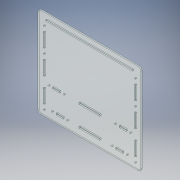
# Autodesk Inventor part: Tapa_Trasera
Saved by Autodesk Inventor 2019 (Build 230136000, 136)
## iProperties
Created: 2020-04-07
Part Number: Tapa_Trasera
Material: Generic
Document SubType Name: Modeling
Designer: Jurgen
Density: 1 g/cm^3
Appearance: Clear
Author: Jurgen
Autodesk Inventor part; units mm, degrees
ref_plane "YZ Plane" through (0, 0, 0) normal (1, 0, 0) x (0, 1, 0)
ref_plane "XZ Plane" through (0, 0, 0) normal (0, 1, 0) x (-1, 0, 0)
ref_plane "XY Plane" through (0, 0, 0) normal (0, 0, 1) x (1, 0, 0)
sketch "Sketch1" plane through (0, 0, 0) normal (0, 0, 1) x (1, 0, 0)
  line L0 (0, 40) -> (0, 0)
  line L1 (0, 40) -> (3.5, 40)
  line L2 (3.5, 40) -> (3.5, 0)
  line L3 (0, 0) -> (3.5, 0)
  line L4 (0, 57) -> (3.5, 57)
  line L5 (3.5, 53) -> (0, 53)
  line L6 (0, -13) -> (3.5, -13)
  line L7 (3.5, -17) -> (0, -17)
  line L8 (0, -30) -> (0, -70)
  line L9 (0, -30) -> (3.5, -30)
  line L10 (3.5, -30) -> (3.5, -70)
  line L11 (0, -70) -> (3.5, -70)
  line L12 (0, -100) -> (0, -140)
  line L13 (3.5, -100) -> (3.5, -140)
  line L14 (0, -100) -> (3.5, -100)
  line L15 (0, -140) -> (3.5, -140)
  line L16 (0, -153) -> (3.5, -153)
  line L17 (3.5, -157) -> (0, -157)
  line L18 (263.5, 57.0001) -> (267, 57.0001)
  line L19 (267, 53.0001) -> (263.5, 53.0001)
  line L20 (263.5, 40.0001) -> (267, 40.0001)
  line L21 (263.5, 40.0001) -> (263.5, 0.0001)
  line L22 (267, 40.0001) -> (267, 0.0001)
  line L23 (263.5, 0.0001) -> (267, 0.0001)
  line L24 (263.5, -12.9999) -> (267, -12.9999)
  line L25 (267, -16.9999) -> (263.5, -16.9999)
  line L26 (263.5, -29.9999) -> (267, -29.9999)
  line L27 (263.5, -29.9999) -> (263.5, -69.9999)
  line L28 (267, -29.9999) -> (267, -69.9999)
  line L29 (263.5, -69.9999) -> (267, -69.9999)
  line L30 (263.5, -99.9999) -> (263.5, -139.9999)
  line L31 (263.5, -99.9999) -> (267, -99.9999)
  line L32 (267, -99.9999) -> (267, -139.9999)
  line L33 (263.5, -139.9999) -> (267, -139.9999)
  line L34 (263.5, -152.9999) -> (267, -152.9999)
  line L35 (267, -156.9999) -> (263.5, -156.9999)
  line L36 (23.5, -149.9999) -> (23.5, -144.9999)
  line L37 (27.5, -144.9999) -> (27.5, -149.9999)
  line L38 (37.5, -144.9999) -> (37.5, -149.9999)
  line L39 (57.5, -144.9999) -> (57.5, -149.9999)
  line L40 (67.5, -149.9999) -> (67.5, -144.9999)
  line L41 (71.5, -144.9999) -> (71.5, -149.9999)
  line L42 (37.5, -144.9999) -> (57.5, -144.9999)
  line L43 (57.5, -149.9999) -> (37.5, -149.9999)
  line L44 (103.5, -144.9999) -> (103.5, -149.9999)
  line L45 (103.5, -144.9999) -> (163.5, -144.9999)
  line L46 (163.5, -149.9999) -> (103.5, -149.9999)
  line L47 (163.5, -144.9999) -> (163.5, -149.9999)
  line L48 (195.5, -149.9999) -> (195.5, -144.9999)
  line L49 (199.5, -144.9999) -> (199.5, -149.9999)
  line L50 (209.5, -144.9999) -> (209.5, -149.9999)
  line L51 (229.5, -144.9999) -> (229.5, -149.9999)
  line L52 (209.5, -144.9999) -> (229.5, -144.9999)
  line L53 (229.5, -149.9999) -> (209.5, -149.9999)
  line L54 (239.5, -149.9999) -> (239.5, -144.9999)
  line L55 (243.5, -144.9999) -> (243.5, -149.9999)
  line L56 (253.5, -84.9999) -> (253.5, -89.9999)
  line L57 (249.5, -89.9999) -> (249.5, -84.9999)
  line L58 (239.5, -84.9999) -> (239.5, -89.9999)
  line L59 (239.5, -84.9999) -> (219.5, -84.9999)
  line L60 (219.5, -84.9999) -> (219.5, -89.9999)
  line L61 (239.5, -89.9999) -> (219.5, -89.9999)
  line L62 (205.5, -89.9999) -> (205.5, -84.9999)
  line L63 (209.5, -84.9999) -> (209.5, -89.9999)
  line L64 (103.5, -84.9999) -> (163.5, -84.9999)
  line L65 (163.5, -89.9999) -> (103.5, -89.9999)
  line L66 (163.5, -84.9999) -> (163.5, -89.9999)
  line L67 (103.5, -84.9999) -> (103.5, -89.9999)
  line L68 (57.5, -89.9999) -> (57.5, -84.9999)
  line L69 (61.5, -84.9999) -> (61.5, -89.9999)
  line L70 (47.5, -84.9999) -> (47.5, -89.9999)
  line L71 (27.5, -84.9999) -> (47.5, -84.9999)
  line L72 (47.5, -89.9999) -> (27.5, -89.9999)
  line L73 (27.5, -84.9999) -> (27.5, -89.9999)
  line L74 (13.5, -89.9999) -> (13.5, -84.9999)
  line L75 (17.5, -84.9999) -> (17.5, -89.9999)
  line L76 (-15, 82) -> (-15, -161.9999)
  arc A0 (-7, 90) -> (-15, 82) centre (-7, 82) ccw
  line L77 (274, 90) -> (-7, 90)
  arc A1 (282, 82) -> (274, 90) centre (274, 82) ccw
  line L78 (282, -161.9999) -> (282, 82)
  arc A2 (-15, -161.9999) -> (-7, -169.9999) centre (-7, -161.9999) ccw
  line L79 (-7, -169.9999) -> (274, -169.9999)
  arc A3 (274, -169.9999) -> (282, -161.9999) centre (274, -161.9999) ccw
  line L80 (1.75, 57) -> (1.75, 53)
  line L81 (1.75, -13) -> (1.75, -17)
  line L82 (1.75, -153) -> (1.75, -157)
  line L83 (23.5, -147.4999) -> (27.5, -147.4999)
  line L84 (67.5, -147.4999) -> (71.5, -147.4999)
  line L85 (195.5, -147.4999) -> (199.5, -147.4999)
  line L86 (239.5, -147.4999) -> (243.5, -147.4999)
  line L87 (265.25, -156.9999) -> (265.25, -152.9999)
  line L88 (13.5, -87.4999) -> (17.5, -87.4999)
  line L89 (57.5, -87.4999) -> (61.5, -87.4999)
  line L90 (205.5, -87.4999) -> (209.5, -87.4999)
  line L91 (249.5, -87.4999) -> (253.5, -87.4999)
  line L92 (265.25, -16.9999) -> (265.25, -12.9999)
  line L93 (265.25, 53.0001) -> (265.25, 57.0001)
  circle A4 centre (1.75, 55) radius 2
  circle A5 centre (1.75, -15) radius 2
  circle A6 centre (1.75, -155) radius 2
  circle A7 centre (25.5, -147.4999) radius 2
  circle A8 centre (69.5, -147.4999) radius 2
  circle A9 centre (197.5, -147.4999) radius 2
  circle A10 centre (241.5, -147.4999) radius 2
  circle A11 centre (265.25, -154.9999) radius 2
  circle A12 centre (15.5, -87.4999) radius 2
  circle A13 centre (59.5, -87.4999) radius 2
  circle A14 centre (207.5, -87.4999) radius 2
  circle A15 centre (251.5, -87.4999) radius 2
  circle A16 centre (265.25, -14.9999) radius 2
  circle A17 centre (265.25, 55.0001) radius 2
  constraints: 188 end point, 42 midpoint, 8 horizontal alignment, 8 point on circle, 7 centre point, 3 tangent, 3 vertical alignment, 22 other
extrude "Extrusion1" add sketch "Sketch1" along normal blind 3.5
sketch "Sketch2" plane through (0, 0, 3.5) normal (0, 0, 1) x (1, 0, 0)
  line L0 (163.5, -84.9999) -> (163.5, -89.9999) construction
  line L1 (163.5, -89.9999) -> (103.5, -89.9999) construction
  line L2 (103.5, -89.9999) -> (103.5, -84.9999) construction
  line L3 (103.5, -84.9999) -> (163.5, -84.9999) construction
  line L4 (103.5, -144.9999) -> (163.5, -144.9999) construction
  line L5 (163.5, -144.9999) -> (163.5, -149.9999) construction
  line L6 (163.5, -149.9999) -> (103.5, -149.9999) construction
  line L7 (103.5, -149.9999) -> (103.5, -144.9999) construction
  line L8 (263.5, -99.9999) -> (267, -99.9999) construction
  line L9 (267, -99.9999) -> (267, -139.9999) construction
  line L10 (267, -139.9999) -> (263.5, -139.9999) construction
  line L11 (263.5, -139.9999) -> (263.5, -99.9999) construction
  line L12 (267, -29.9999) -> (267, -69.9999) construction
  line L13 (267, -69.9999) -> (263.5, -69.9999) construction
  line L14 (263.5, -69.9999) -> (263.5, -29.9999) construction
  line L15 (263.5, -29.9999) -> (267, -29.9999) construction
  line L16 (267, 40.0001) -> (267, 0.0001) construction
  line L17 (267, 0.0001) -> (263.5, 0.0001) construction
  line L18 (263.5, 0.0001) -> (263.5, 40.0001) construction
  line L19 (263.5, 40.0001) -> (267, 40.0001) construction
  line L20 (0, -100) -> (3.5, -100) construction
  line L21 (3.5, -100) -> (3.5, -140) construction
  line L22 (3.5, -140) -> (0, -140) construction
  line L23 (0, -140) -> (0, -100) construction
  line L24 (0, -30) -> (3.5, -30) construction
  line L25 (3.5, -30) -> (3.5, -70) construction
  line L26 (3.5, -70) -> (0, -70) construction
  line L27 (0, -70) -> (0, -30) construction
  line L28 (0, 40) -> (3.5, 40) construction
  line L29 (3.5, 40) -> (3.5, 0) construction
  line L30 (3.5, 0) -> (0, 0) construction
  line L31 (0, 0) -> (0, 40) construction
  line L32 (47.5, -89.9999) -> (27.5, -89.9999) construction
  line L33 (27.5, -89.9999) -> (27.5, -84.9999) construction
  line L34 (27.5, -84.9999) -> (47.5, -84.9999) construction
  line L35 (47.5, -84.9999) -> (47.5, -89.9999) construction
  line L36 (239.5, -89.9999) -> (219.5, -89.9999) construction
  line L37 (219.5, -89.9999) -> (219.5, -84.9999) construction
  line L38 (219.5, -84.9999) -> (239.5, -84.9999) construction
  line L39 (239.5, -84.9999) -> (239.5, -89.9999) construction
  line L40 (209.5, -144.9999) -> (229.5, -144.9999) construction
  line L41 (229.5, -144.9999) -> (229.5, -149.9999) construction
  line L42 (229.5, -149.9999) -> (209.5, -149.9999) construction
  line L43 (209.5, -149.9999) -> (209.5, -144.9999) construction
  line L44 (37.5, -144.9999) -> (57.5, -144.9999) construction
  line L45 (57.5, -144.9999) -> (57.5, -149.9999) construction
  line L46 (57.5, -149.9999) -> (37.5, -149.9999) construction
  line L47 (37.5, -149.9999) -> (37.5, -144.9999) construction
  circle A0 centre (265.25, 55.0001) radius 2 construction
  circle A1 centre (265.25, -14.9999) radius 2 construction
  circle A2 centre (251.5, -87.4999) radius 2 construction
  circle A3 centre (207.5, -87.4999) radius 2 construction
  circle A4 centre (59.5, -87.4999) radius 2 construction
  circle A5 centre (15.5, -87.4999) radius 2 construction
  circle A6 centre (265.25, -154.9999) radius 2 construction
  circle A7 centre (241.5, -147.4999) radius 2 construction
  circle A8 centre (197.5, -147.4999) radius 2 construction
  circle A9 centre (69.5, -147.4999) radius 2 construction
  circle A10 centre (25.5, -147.4999) radius 2 construction
  circle A11 centre (1.75, -155) radius 2 construction
  circle A12 centre (1.75, -15) radius 2 construction
  circle A13 centre (1.75, 55) radius 2 construction
  line L48 (-15, 82) -> (-15, -161.9999) construction
  arc A14 (-15, -161.9999) -> (-7, -169.9999) centre (-7, -161.9999) ccw construction
  line L49 (-7, -169.9999) -> (274, -169.9999) construction
  arc A15 (274, -169.9999) -> (282, -161.9999) centre (274, -161.9999) ccw construction
  line L50 (282, -161.9999) -> (282, 82) construction
  arc A16 (282, 82) -> (274, 90) centre (274, 82) ccw construction
  line L51 (274, 90) -> (-7, 90) construction
  arc A17 (-7, 90) -> (-15, 82) centre (-7, 82) ccw construction
  line L52 (-15, 82) -> (-15, 90) construction
  line L53 (-15, 90) -> (-7, 90) construction
  line L54 (-15.8616, 90) -> (7.6384, 90) construction
  line L55 (7.6384, 90) -> (7.6384, 73.5) construction
  line L56 (7.6384, 73.5) -> (-15.8616, 73.5) construction
  line L57 (-15.8616, 73.5) -> (-15.8616, 90) construction
  line L58 (7.6384, 73.5) -> (257.6384, 73.5)
  line L59 (257.6384, 73.5) -> (257.6384, 70)
  line L60 (257.6384, 70) -> (7.6384, 70)
  line L61 (7.6384, 70) -> (7.6384, 73.5)
  dimension "d2" = 23.5
  dimension "d3" = 16.5
  dimension "d4" = 250
  dimension "d5" = 3.5
  constraints: 20 end point, 4 parallel, 3 perpendicular, 2 horizontal, 1 tangent, 1 vertical
  measures "d2" distance of L55.end L56.end
  measures "d3" distance of L54.end L55.end
  measures "d4" distance of L59.end L60.end
  measures "d5" distance of L58.end L59.end
extrude "Extrusion2" cut sketch "Sketch2" against normal blind 3.5
body "Solid1"
